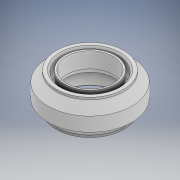
# Autodesk Inventor part: Internal_V-groove_Bearing
Saved by Autodesk Inventor 2020.2 (Build 242310000, 310)
## iProperties
Created: 2020-04-04
Part Number: Internal_V-groove_Bearing
Material: Generic
Document SubType Name: Modeling
Designer: rah75
Density: 1 g/cm^3
Appearance: Default
Author: rah75
Autodesk Inventor part; units mm, degrees
ref_plane "YZ Plane" through (0, 0, 0) normal (1, 0, 0) x (0, 1, 0)
ref_plane "XZ Plane" through (0, 0, 0) normal (0, 1, 0) x (-1, 0, 0)
ref_plane "XY Plane" through (0, 0, 0) normal (0, 0, 1) x (1, 0, 0)
sketch "Sketch1" plane through (0, 0, 0) normal (0, 0, 1) x (1, 0, 0)
  line L0 (0, -0.4401) -> (0, 0.4401)
  line L1 (-8.125, -0.5) -> (-6.95, -0.5)
  line L2 (-6.95, -0.5) -> (-6.95, 0.5)
  line L3 (-6.95, 0.5) -> (-8.125, 0.5)
  line L4 (-8.125, 0.5) -> (-8.125, -0.5)
  line L5 (-8.125, -0.5) -> (-6.95, 0.5) construction
  line L6 (-6.95, -0.5) -> (-8.125, 0.5) construction
  line L7 (-9.625, 5) -> (-8.125, 5)
  line L8 (-8.125, 5) -> (-8.125, -5)
  line L9 (-8.125, -5) -> (-9.625, -5)
  line L10 (-9.625, -5) -> (-9.625, 5)
  line L11 (-9.625, 5) -> (-8.125, -5) construction
  line L12 (-8.125, 5) -> (-9.625, -5) construction
  line L13 (-9.625, -4.375) -> (-12, -2)
  line L14 (-12, -2) -> (-12, 2)
  line L15 (-12, 2) -> (-9.625, 4.375)
  line L16 (-8, 0.5) -> (8, 0.5) construction
  line L17 (8, 0.5) -> (8, 5.5) construction
  line L18 (8, 5.5) -> (-8, 5.5) construction
  line L19 (-8, 5.5) -> (-8, 0.5) construction
  line L20 (-8, 0.5) -> (8, 5.5) construction
  line L21 (8, 0.5) -> (-8, 5.5) construction
  line L22 (-17, -3) -> (-11, -3) construction
  line L23 (-11, -3) -> (-11, 3) construction
  line L24 (-11, 3) -> (-17, 3) construction
  line L25 (-17, 3) -> (-17, -3) construction
  line L26 (-17, -3) -> (-11, 3) construction
  line L27 (-11, -3) -> (-17, 3) construction
  point P0 (0, 0)
  point P1 (0, 0)
  point P2 (-7.5375, 0)
  point P3 (-8.875, 0)
  point P4 (-12, 0)
  point P5 (-7.5375, 0)
  point P6 (-8.875, 0)
  point P7 (0, 3)
  point P8 (0, 3)
  point P9 (-14, 0)
  point P10 (-8.125, 0.5)
  point P11 (-8.125, -0.5)
  dimension "d0" = 13.9
  dimension "d1" = 16.25
  dimension "d2" = 10
  dimension "d3" = 16
  dimension "d4" = 5
  dimension "d5" = 5.5
  dimension "d6" = 45
  dimension "d7" = 4
  dimension "d8" = 2.375
  dimension "d9" = 1.5
  dimension "d10" = 6
  dimension "d11" = 6
  dimension "d12" = 22
  constraints: 56 end point, 13 midpoint, 8 parallel, 5 perpendicular, 4 horizontal, 4 point on line, 3 horizontal alignment, 2 collinear, 2 vertical, 1 coincident, 1 vertical alignment
  measures "d0" diameter of L2 L0
  measures "d1" diameter of L8 L0
  measures "d2" distance of L7.end L8.end
  measures "d3" distance of L18.end L17.end
  measures "d4" distance of L17.end L16.end
  measures "d5" distance from line of point (0, 0) L18
  measures "d6" angle of L10 L15
  measures "d7" distance of L13.end L14.end
  measures "d8" distance between parallel lines of L10 L14
  measures "d9" distance of L7.start L7.end
  measures "d10" distance of L24.end L23.end
  measures "d11" distance of L23.end L22.end
  measures "d12" diameter of L23 L0
revolve "Revolution1" add sketch "Sketch1" angle 360 about axis through (0, -0.4401, 0) along (0, 1, 0)
chamfer "Chamfer1" distance 0.5 angle 45 2 edges at (8.125, 5, 0) (8.125, -5, 0)
sketch "Sketch2" plane through (0, 0.5, 0) normal (0, 1, 0) x (1, 0, 0)
  circle A0 centre (0, 0) radius 6.95 construction
  circle A1 centre (0, 0) radius 7.2
  circle A2 centre (0, 0) radius 6.7
  point P0 (0, 0)
  dimension "d17" = 0.25
  dimension "d18" = 0.25
  constraints: 2 centre point
  measures "d17" radial gap between concentric circles of A0 A1
  measures "d18" radial gap between concentric circles of A0 A2
extrude "Extrusion1" add sketch "Sketch2" along normal up to surface (4.5 mm away)
body "Solid1"
